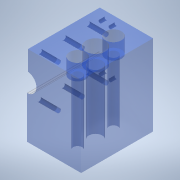
# Autodesk Inventor part: zgalvo_to_newport_stage
Saved by Autodesk Inventor 2022 (Build 260153000, 153)
## iProperties
Created: 2015-03-27
Part Number: zgalvo_to_newport_stage
Material: ALUMINUM, 6061-T651
Document SubType Name: Modeling
Designer: legantw
Density: 2.7 g/cm^3
Appearance: Clear - Blue
Catalog Web Link: MPFI custom
Description: zgalvo_to_optisigma_stage
Project: P-303502
Vendor: HHMI: JRC - JET
Stock Number: J007526
ALTERED ITEM PART NUMBER: N/A
ALTERED ITEM VENDOR: N/A
ALTERED ITEM DESCRIPTION: N/A
DESIGN DEPARTMENT: HHMI: JRC - ID&F
LAB/DEPT: BETZIG (LAB)
REQUESTING SCIENTIST: BETZIG, ERIC
SPECIAL FINISH: ANODIZE PER MIL-A-8625F, TYPE II, CLASS 2 (BLACK)
SURFACE ROUGHNESS: 32 Ra
Author: legantw
Revision Number: 0
Autodesk Inventor part; units mm, degrees
note: some values were not read from the file. Chosen so that the rebuilt part matches the saved one: direction of "Emboss1".
ref_plane "YZ Plane" through (0, 0, 0) normal (1, 0, 0) x (0, 1, 0)
ref_plane "XZ Plane" through (0, 0, 0) normal (0, 1, 0) x (-1, 0, 0)
ref_plane "XY Plane" through (0, 0, 0) normal (0, 0, 1) x (1, 0, 0)
sketch "Sketch1" plane through (0, 0, 0) normal (0, 0, 1) x (1, 0, 0)
  line L0 (-15.5, 18) -> (19.5, 18)
  line L1 (19.5, 18) -> (19.5, -18)
  line L2 (19.5, -18) -> (-15.5, -18)
  line L3 (-15.5, -18) -> (-15.5, 18)
  point P0 (0, 0)
  dimension "d0" = 35
  dimension "d1" = 36
  dimension "d2" = 18
  dimension "d3" = 15.5
  constraints: 8 end point, 2 parallel, 1 horizontal, 1 perpendicular
  measures "d0" distance of L0.start L0.end
  measures "d1" distance of L0.end L1.end
  measures "d2" distance from line of L0 point (0, 0)
  measures "d3" distance from line of L3 point (0, 0)
extrude "Extrusion1" add sketch "Sketch1" along normal blind 8
sketch "Sketch2" plane through (0, 0, 8) normal (0, 0, 1) x (1, 0, 0)
  line L0 (-15.5, 18) -> (19.5, 18)
  line L1 (19.5, 18) -> (19.5, -18)
  line L2 (19.5, -18) -> (-15.5, -18)
  line L3 (-15.5, -18) -> (-15.5, 18)
  line L4 (-15.5, -18) -> (-15.5, 18) projected
  line L5 (19.5, 18) -> (19.5, -18) projected
  line L6 (-15.5, 18) -> (19.5, 18) projected
  line L7 (19.5, -18) -> (-15.5, -18) projected
  line L8 (19.5, -18) -> (19.5, 18)
  point P0 (0, 0)
  dimension "d70" = 0
  dimension "d165" = 0
  constraints: 10 end point, 5 point on line, 2 parallel, 2 perpendicular, 1 horizontal
  measures "d70" distance between parallel lines of L4 L3
  measures "d165" distance between parallel lines of L1 L8
extrude "Extrusion2" add sketch "Sketch2" along normal blind 22.5
sketch "Sketch3" plane through (-15.5, -18, 0) normal (0, -1, 0) x (1, 0, 0)
  line L0 (7.85, 30.5) -> (7.35, 30.5)
  line L1 (7.85, 30.5) -> (8.35, 30.5)
  line L2 (35, 0) -> (0, 0) projected
  arc A0 (7.35, 20.7234) -> (8.35, 20.7234) centre (7.85, 16) ccw
  line L3 (7.35, 30.5) -> (7.35, 20.7234)
  line L4 (8.35, 30.5) -> (8.35, 20.7234)
  line L5 (35, 0) -> (35, 30.5) projected
  line L6 (35, 30.5) -> (0, 30.5) projected
  line L7 (0, 0) -> (0, 30.5) projected
  point P0 (15.5, 0)
  dimension "d16" = 0.5
  dimension "d17" = 0.5
  dimension "d63" = 9.4996
  dimension "d65" = 16
  dimension "d105" = 1
  dimension "d188" = 7.85
  dimension "d189" = 0.5
  constraints: 8 end point, 2 point on circle, 2 point on line, 1 centre point, 1 parallel, 1 vertical
  measures "d16" distance of L0.start L0.end
  measures "d17" distance of L0.start L1.end
  measures "d63" diameter of A0
  measures "d65" distance from line of L2 A0.centre
  measures "d105" distance of L3.end L4.end
  measures "d188" distance from line of L7 A0.centre
  measures "d189" distance from line of A0.centre L4
emboss "Emboss1" sketch "Sketch3" operation cut depth 50 direction (0, 1, 0) contours L1 L4 A0 L3 L0
sketch "Sketch13" plane through (0, 0, 0) normal (0, 0, -1) x (-1, 0, 0)
  line L0 (-13, -5.3) -> (11, -5.3)
  line L1 (15.5, 18) -> (-19.5, 18) projected
  line L2 (-19.5, 18) -> (-19.5, -18) projected
  line L3 (-19.5, -18) -> (15.5, -18) projected
  line L4 (15.5, -18) -> (15.5, 18) projected
  line L5 (-19.5, 18) -> (-19.5, -18) projected
  line L6 (-19.5, -5.3) -> (15.5, -5.3)
  point P0 (0, 0)
  dimension "d190" = 12.7
  constraints: 4 end point, 3 point on line, 1 collinear
  measures "d190" distance between parallel lines of L3 L0
extrude "Extrusion5" [suppressed]
sketch "Sketch14" plane through (-15.5, -5.3, 0) normal (0, 1, 0) x (1, 0, 0)
  line L0 (0, 32) -> (35, 32) projected
  line L1 (35, 0) -> (35, 32) projected
  point P0 (15.5, 0)
  point P1 (9.5, 30)
  point P2 (28, 30)
  point P3 (32.75, 16)
  dimension "d109" = 2
  dimension "d110" = 2
  dimension "d111" = 2.25
  dimension "d112" = 9.5
  dimension "d113" = 7
  dimension "d114" = 16
  measures "d109" distance from line of L0 point (9.5, 30)
  measures "d110" distance from line of L0 point (28, 30)
  measures "d111" distance from line of L1 point (32.75, 16)
  measures "d112" horizontal distance of L0.start point (9.5, 30)
  measures "d113" horizontal distance of L0.end point (28, 30)
  measures "d114" vertical distance of L0.end point (32.75, 16)
hole "Press fit for D2mm_L5mm Dowel - pin to protrude 2mm" [suppressed]
sketch "Sketch21" plane through (0, 0, 0) normal (0, 0, -1) x (-1, 0, 0)
  circle A0 centre (-3.75, 0.2) radius 3
  circle A1 centre (-3.75, 0.2) radius 3 construction
  point P0 (0, 0)
  dimension "d185" = 6
  constraints: 2 centre point, 1 coincident, 2 other
  measures "d185" diameter of A0
sketch "Sketch22" plane through (-15.5, -18, 30.5) normal (-1, 0, 0) x (0, 0, 1)
  line L0 (-30.5, 36) -> (0, 36) projected
  line L1 (-30.5, 0) -> (-30.5, 36) projected
  line L2 (-30.5, 0) -> (0, 0) projected
  line L3 (0, 0) -> (0, 36) projected
  point P0 (-30.5, 18)
  point P1 (-4, 30)
  point P2 (-4, 18)
  point P3 (-4, 6)
  dimension "d191" = 4
  dimension "d192" = 4
  dimension "d193" = 4
  dimension "d194" = 6
  dimension "d195" = 6
  dimension "d196" = 18
  measures "d191" distance from line of L3 point (-4, 30)
  measures "d192" distance from line of L3 point (-4, 18)
  measures "d193" distance from line of L3 point (-4, 6)
  measures "d194" distance from line of L2 point (-4, 6)
  measures "d195" distance from line of L0 point (-4, 30)
  measures "d196" distance from line of L0 point (-4, 18)
hole "CBore for M2.5 screw" [suppressed]
sketch "Sketch24" plane through (-7.65, -18, 16) normal (0, -1, 0) x (1, 0, 0)
  circle A0 centre (21.4, -42.5) radius 0.7835
  circle A1 centre (21.4, -22.5) radius 0.7835
  circle A2 centre (1.4, -42.5) radius 0.7835
  circle A3 centre (1.4, -22.5) radius 0.7835
  point P0 (7.65, -16)
  constraints: 4 centre point, 8 other
hole "CBore for M2 screw" [suppressed]
sketch "Sketch25" plane through (-7.65, -18, 16) normal (0, -1, 0) x (1, 0, 0)
  line L0 (-0.5, 4.7234) -> (-0.5, 14.5) projected
  line L1 (-0.5, 14.5) -> (-7.85, 14.5) projected
  line L2 (-7.85, -16) -> (-7.85, 14.5) projected
  line L3 (27.15, -16) -> (27.15, 14.5) projected
  line L4 (27.15, 14.5) -> (0.5, 14.5) projected
  line L5 (0.5, 14.5) -> (0.5, 4.7234) projected
  arc A0 (-0.5, 4.7234) -> (0.5, 4.7234) centre (0, 0) ccw projected
  line L6 (27.15, -48) -> (-7.85, -48) projected
  circle A1 centre (1.4, -42.5) radius 2.2 projected
  circle A2 centre (21.4, -42.5) radius 1.2 projected
  line L7 (1.4, -42.5) -> (21.4, -42.5) construction
  line L8 (11.4, -42.5) -> (11.4, 14.5) construction
  line L9 (0.5, 14.5) -> (27.15, 14.5) projected
  line L10 (27.15, -16) -> (-7.85, -16) projected
  point P0 (7.65, -16)
  point P1 (11.4, -23)
  point P2 (11.4, -40)
  constraints: 4 end point, 3 point on line, 1 horizontal, 1 midpoint, 1 perpendicular
hole "Threaded hole for M2 screw" [suppressed]
sketch "Sketch27" plane through (-15.5, 18, 0) normal (0, 1, 0) x (1, 0, 0)
  arc A0 (8.35, -20.7234) -> (7.35, -20.7234) centre (7.85, -16) ccw projected
  line L0 (7.35, -30.5) -> (7.35, -20.7234) projected
  arc A1 (8.35, -20.7234) -> (7.35, -20.7234) centre (7.85, -16) ccw projected
  line L1 (8.35, -20.7234) -> (8.35, -30.5) projected
  line L2 (8.35, -30.5) -> (35, -30.5) projected
  line L3 (35, 0) -> (35, -30.5) projected
  line L4 (0, 0) -> (35, 0) projected
  line L5 (0, 0) -> (0, -30.5) projected
  line L6 (0, -30.5) -> (7.35, -30.5) projected
  line L7 (7.85, -16) -> (7.85, -30.5)
  line L8 (7.85, -30.5) -> (0, -30.5)
  line L9 (0, -30.5) -> (0, 0)
  line L10 (0, 0) -> (7.85, 0)
  line L11 (7.85, 0) -> (7.85, -16)
  point P0 (15.5, 0)
  constraints: 10 end point, 2 perpendicular, 2 point on line, 1 collinear, 1 vertical
extrude "Extrusion7" cut sketch "Sketch27" against normal through all contours L11 L7 L8 L0 A0 | A0 L0 L6 L5 L4 L11
sketch "Sketch23" plane through (-7.65, -18, 20.7234) normal (-1, 0, 0) x (0, 0, 1)
  line L0 (0, 0) -> (-9.4732, 0) construction
  line L1 (-9.4732, 36) -> (0, 36) construction
  line L2 (-4.7366, 0) -> (-4.7366, 36) construction
  point P0 (-20.7234, 18)
  point P1 (5.7766, 30)
  point P2 (5.7766, 18)
  point P3 (5.7766, 6)
  point P4 (-15.2498, 30)
  point P5 (-15.2498, 18)
  point P6 (-15.2498, 6)
  point P7 (5.7766, 30)
  point P8 (5.7766, 18)
  point P9 (5.7766, 6)
  dimension "d227" = 10.5132
  dimension "d228" = 10.5132
  dimension "d229" = 10.5132
  dimension "d230" = 10.5132
  dimension "d231" = 10.5132
  dimension "d232" = 10.5132
  dimension "d233" = 6
  dimension "d234" = 6
  dimension "d235" = 18
  dimension "d236" = 30
  dimension "d237" = 18
  dimension "d238" = 30
  constraints: 3 coincident, 2 end point, 2 midpoint
  measures "d227" distance from line of L2 point (5.777, 30)
  measures "d228" distance from line of L2 point (5.777, 18)
  measures "d229" distance from line of L2 point (5.777, 6)
  measures "d230" distance from line of point (-15.25, 6) L2
  measures "d231" distance from line of L2 point (-15.25, 18)
  measures "d232" distance from line of L2 point (-15.25, 30)
  measures "d233" distance from line of L1 point (-15.25, 30)
  measures "d234" distance from line of L1 point (5.777, 30)
  measures "d235" distance from line of L1 point (5.777, 18)
  measures "d236" distance from line of L1 point (5.777, 6)
  measures "d237" distance from line of L1 point (-15.25, 18)
  measures "d238" distance from line of L1 point (-15.25, 6)
hole "Threaded hole for M2.5 screw" at (-7.65, 12, 26.5) at (-7.65, 0, 26.5) at (-7.65, -12, 26.5) at (-7.65, 12, 5.4736) at (-7.65, 0, 5.4736) at (-7.65, -12, 5.4736) direction (1, 0, 0) diameter 2.013 depth 10 tip angle 118 thread size "M2.5x0.45" class "6H" standard "ANSI Metric M Profile"
sketch "Sketch29" plane through (19.5, 18, 30.5) normal (0, 1, 0) x (1, 0, 0)
  arc A0 (-26.65, 9.7766) -> (-27.15, 19.2498) centre (-27.15, 14.5) ccw projected
  point P0 (-19.5, 30.5)
  point P1 (-23.5, 3)
  point P2 (-18.5, 3)
  point P3 (-23.5, 26)
  point P4 (-18.5, 26)
  dimension "d241" = 11.5
  dimension "d242" = 11.5
  dimension "d243" = 11.5
  dimension "d244" = 11.5
  dimension "d245" = 3.65
  dimension "d246" = 3.65
  dimension "d247" = 8.65
  dimension "d248" = 8.65
  measures "d241" vertical distance of point (-23.5, 3) A0.centre
  measures "d242" vertical distance of A0.centre point (-18.5, 3)
  measures "d243" vertical distance of A0.centre point (-23.5, 26)
  measures "d244" vertical distance of A0.centre point (-18.5, 26)
  measures "d245" horizontal distance of A0.centre point (-23.5, 26)
  measures "d246" horizontal distance of A0.centre point (-23.5, 3)
  measures "d247" horizontal distance of A0.centre point (-18.5, 3)
  measures "d248" horizontal distance of A0.centre point (-18.5, 26)
hole "Hole18" at (-4, 18, 27.5) at (1, 18, 27.5) at (-4, 18, 4.5) at (1, 18, 4.5) direction (0, -1, 0) diameter 1.567 depth 3 tip angle 118 thread size "M2x0.4" class "6H" standard "ANSI Metric M Profile"
sketch "Sketch31" plane through (0, 0, 0) normal (0, 0, -1) x (-1, 0, 0)
  line L0 (7.65, 18) -> (-19.5, 18) projected
  line L1 (7.65, -18) -> (7.65, 18) projected
  line L2 (-19.5, 18) -> (7.65, 18)
  line L3 (7.65, 18) -> (7.65, -18)
  line L4 (7.65, -18) -> (-19.5, -18)
  line L5 (-19.5, -18) -> (-19.5, 18)
  line L6 (-19.5, 18) -> (7.65, 18)
  line L7 (7.65, 18) -> (7.65, -18)
  line L8 (7.65, -18) -> (-19.5, -18)
  line L9 (-19.5, -18) -> (-19.5, 18)
  point P0 (0, 0)
  constraints: 16 end point, 4 parallel, 2 horizontal, 2 perpendicular
extrude "Extrusion8" add sketch "Sketch31" along normal blind 9.9003
hole "Hole19" [suppressed]
sketch "Sketch30" plane through (0, 0, 30.5) normal (0, 0, 1) x (1, 0, 0)
  circle A0 centre (8.5, 0.2) radius 3
  line L0 (19.5, 18) -> (19.5, -18) projected
  line L1 (-7.15, 18) -> (19.5, 18) projected
  circle A1 centre (8.5, 9.1803) radius 1.1674
  circle A2 centre (8.5, -8.7803) radius 1.2033
  point P0 (0, 0)
  dimension "d263" = 6
  dimension "d264" = 11
  dimension "d265" = 17.8
  dimension "d273" = 8.9803
  dimension "d274" = 8.9803
  constraints: 3 centre point
  measures "d263" diameter of A0
  measures "d264" distance from line of L0 A0.centre
  measures "d265" distance from line of L1 A0.centre
  measures "d273" distance of A0.centre A1.centre
  measures "d274" distance of A0.centre A2.centre
hole "Hole20" at (8.5, 0.2, 30.5) direction (0, 0, -1) diameter 6.756 end through all counterbore diameter 9.652 counterbore depth 8 clearance for "Hex Head Bolt" size "1/4" standard "Ansi Unified Screw Threads"
hole "Hole21" at (8.5, 9.1803, 30.5) direction (0, 0, -1) diameter 4.496 end through all counterbore diameter 7.938 counterbore depth 8 clearance for "Socket Head Cap Screw" size "#8" standard "Ansi Unified Screw Threads"
hole "Hole22" at (8.5, -8.7803, 30.5) direction (0, 0, -1) diameter 4.496 end through all counterbore diameter 7.938 counterbore depth 8 clearance for "Socket Head Cap Screw" size "#8" standard "Ansi Unified Screw Threads"
equation "\"d2\" = 0.5 * d1"
equation "\"d230\" = d229"
equation "\"d231\" = d228"
equation "\"d232\" = d227"
equation "\"d233\" = d234"
equation "\"d237\" = d235"
equation "\"d238\" = d236"
body "Solid1"
